Autodesk Fusion 360 part; units mm, degrees
(part 2 of 2)
  line L359 (-153.6501, -64.1628) -> (-153.6501, 86.0492)
  line L360 (173.4959, -17.9288) -> (186.4959, -17.9288)
  line L361 (186.4959, -17.9288) -> (186.4959, -30.9288)
  line L362 (186.4959, -30.9288) -> (173.4959, -30.9288)
  line L363 (173.4959, -30.9288) -> (173.4959, -17.9288)
  circle A356 centre (207.0639, 80.5492) radius 1.45
  circle A357 centre (-148.1501, 80.5492) radius 1.45
  circle A358 centre (-148.1501, -58.6628) radius 1.45
  circle A359 centre (207.0639, -58.6628) radius 1.45
  dimension "d1" = 366.214
  dimension "d2" = 150.212
  dimension "d3" = 16.317
  dimension "d4" = 21.381
  dimension "d5" = 13
  dimension "d6" = 13
  dimension "d7" = 26.068
  dimension "d8" = 33.234
  dimension "d9" = 2.9
  dimension "d10" = 5.5
  dimension "d11" = 5.5
  dimension "d12" = 2.9
  dimension "d13" = 5.5
  dimension "d14" = 5.5
  dimension "d15" = 2.9
  dimension "d16" = 5.5
  dimension "d17" = 5.5
  dimension "d18" = 2.9
  dimension "d19" = 5.5
  dimension "d20" = 5.5
  constraint horizontal L356
  constraint vertical L357
  constraint horizontal L358
  constraint vertical L359
  constraint horizontal L360
  constraint vertical L361
  constraint horizontal L362
  constraint vertical L363
  measures "d1" distance of L357 L359
  measures "d2" distance of L356 L358
  measures "d3" distance of L310 L359
  measures "d4" distance of L309 L358
  measures "d5" distance of L360 L362
  measures "d6" distance of L361 L363
  measures "d7" distance of L357 L361
  measures "d8" distance of L358 L362
  measures "d9" diameter of A359
  measures "d10" distance of L357 A359.centre
  measures "d11" distance of L358 A359.centre
  measures "d12" diameter of A356
  measures "d13" distance of L357 A356.centre
  measures "d14" distance of L356 A356.centre
  measures "d15" diameter of A358
  measures "d16" distance of L358 A358.centre
  measures "d17" distance of L359 A358.centre
  measures "d18" diameter of A357
  measures "d19" distance of L356 A357.centre
  measures "d20" distance of L359 A357.centre
extrude "Extrude1" add sketch "Sketch1" along normal blind 3
fillet "Fillet1" radius 7 4 edges at (212.5639, -64.1628, 1.5) (212.5639, 86.0492, 1.5) (-153.6501, 86.0492, 1.5) (-153.6501, -64.1628, 1.5)
